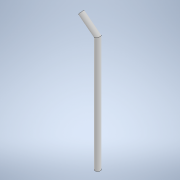
# Autodesk Inventor part: feedthroughpipe
Saved by Autodesk Inventor 2020 (Build 240168000, 168)
## iProperties
Created: 2019-07-26
Part Number: feedthroughpipe
Material: Generic
Document SubType Name: Modeling
Designer: ColinP
Density: 1 g/cm^3
Appearance: Default
Author: ColinP
Autodesk Inventor part; units mm, degrees
ref_plane "YZ Plane" through (0, 0, 0) normal (1, 0, 0) x (0, 1, 0)
ref_plane "XZ Plane" through (0, 0, 0) normal (0, 1, 0) x (-1, 0, 0)
ref_plane "XY Plane" through (0, 0, 0) normal (0, 0, 1) x (1, 0, 0)
sketch "Sketch1" plane through (0, 0, 0) normal (0, 1, 0) x (-1, 0, 0)
  circle A0 centre (0, 0) radius 2.286
  circle A1 centre (0, 0) radius 3.175
  dimension "d0" = 4.572
  dimension "d1" = 6.35
  constraints: 2 centre point, 2 coincident
  measures "d0" diameter of A0
  measures "d1" diameter of A1
sketch "Sketch2" plane through (0, 0, 0) normal (0, 0, 1) x (1, 0, 0)
  line L0 (0, 0) -> (0, 92.964)
  line L1 (0, 0) -> (92.964, 0) construction
  line L2 (0, 92.964) -> (0, 141.224)
  line L3 (0, 141.224) -> (-20.0427, 156.8268)
  line L4 (0, 141.224) -> (25.4, 141.224) construction
  dimension "d2" = 92.964
  dimension "d3" = 90
  dimension "d4" = 48.26
  dimension "d5" = 25.4
  dimension "d6" = 142.1
  constraints: 10 end point, 2 equal length, 2 horizontal, 2 vertical
  measures "d2" distance of L0.start L0.end
  measures "d3" angle of L1 L0
  measures "d4" distance of L0.end L2.end
  measures "d5" distance of L2.end L3.end
  measures "d6" angle of L4 L3
sweep "Sweep1" add profiles "Sketch1" path "Sketch2"
body "Solid1"
